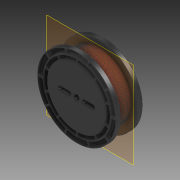
# Autodesk Inventor part: 1240_Wire Spool and Wire
Saved by Autodesk Inventor 2020 (Build 240168000, 168)
## iProperties
Created: 2019-09-24
Part Number: 1240_Wire Spool and Wire
Material: Generic
Document SubType Name: Modeling
Designer: MPI
Density: 1 g/cm^3
Appearance: Default
Author: MPI
Autodesk Inventor part; units mm, degrees
ref_plane "YZ Plane" through (0, 0, 0) normal (1, 0, 0) x (0, 1, 0)
ref_plane "XZ Plane" through (0, 0, 0) normal (0, 1, 0) x (-1, 0, 0)
ref_plane "XY Plane" through (0, 0, 0) normal (0, 0, 1) x (1, 0, 0)
sketch "Sketch1" plane through (0, 0, 0) normal (0, 0, 1) x (1, 0, 0)
  circle A0 centre (0, 0) radius 303
  circle A1 centre (0, 0) radius 20
  line L0 (-125, 15) -> (-57.5, 15)
  line L1 (-57.5, -15) -> (-125, -15)
  line L2 (57.5, 15) -> (125, 15)
  line L3 (125, -15) -> (57.5, -15)
  arc A2 (-57.5, -15) -> (-57.5, 15) centre (-57.5, 0) ccw
  arc A3 (57.5, 15) -> (57.5, -15) centre (57.5, 0) ccw
  arc A4 (125, -15) -> (125, 15) centre (125, 0) ccw
  arc A5 (-125, 15) -> (-125, -15) centre (-125, 0) ccw
  dimension "d0" = 606
  dimension "d12" = 40
  dimension "d15" = 30
  dimension "d16" = 30
  dimension "d17" = 15
  dimension "d18" = 15
  dimension "d19" = 115
  dimension "d20" = 57.5
  dimension "d21" = 250
  dimension "d22" = 125
  constraints: 8 end point, 8 point on circle, 6 centre point, 2 coincident, 2 horizontal, 2 parallel
  measures "d0" diameter of A0
  measures "d12" diameter of A1
  measures "d15" distance of L0.end L1.start
  measures "d16" distance of L3.end L2.start
  measures "d17" distance from line of L3 point (0, 0)
  measures "d18" distance from line of L1 point (0, 0)
  measures "d19" distance of A3.centre A2.centre
  measures "d20" distance of point (0, 0) A2.centre
  measures "d21" distance of A4.centre A5.centre
  measures "d22" distance of point (0, 0) A5.centre
extrude "Extrusion1" add sketch "Sketch1" along normal blind 35
sketch "Sketch2" plane through (0, 0, 35) normal (0, 0, 1) x (1, 0, 0)
  circle A0 centre (0, 0) radius 243
  circle A1 centre (0, 0) radius 20
  arc A2 (-125, 15) -> (-125, -15) centre (-125, 0) ccw projected
  arc A3 (-125, 15) -> (-125, -15) centre (-125, 0) ccw
  arc A4 (-57.5, -15) -> (-57.5, 15) centre (-57.5, 0) ccw projected
  arc A5 (-57.5, -15) -> (-57.5, 15) centre (-57.5, 0) ccw
  arc A6 (57.5, 15) -> (57.5, -15) centre (57.5, 0) ccw projected
  arc A7 (57.5, 15) -> (57.5, -15) centre (57.5, 0) ccw
  arc A8 (125, -15) -> (125, 15) centre (125, 0) ccw projected
  arc A9 (125, -15) -> (125, 15) centre (125, 0) ccw
  line L0 (-125, 15) -> (-57.5, 15) projected
  line L1 (-57.5, -15) -> (-125, -15) projected
  line L2 (-125, 15) -> (-57.5, 15)
  line L3 (-57.5, -15) -> (-125, -15)
  line L4 (125, -15) -> (57.5, -15) projected
  line L5 (57.5, 15) -> (125, 15)
  line L6 (125, -15) -> (57.5, -15)
  point P0 (125, 15)
  dimension "d3" = 486
  dimension "d14" = 40
  constraints: 9 end point, 9 point on circle, 6 centre point, 6 coincident, 2 horizontal, 2 parallel
  measures "d3" diameter of A0
  measures "d14" diameter of A1
extrude "Extrusion2" add sketch "Sketch2" along normal blind 134 separate body
sketch "Sketch3" plane through (0, 0, 169) normal (0, 0, 1) x (1, 0, 0)
  circle A0 centre (0, 0) radius 303
  circle A1 centre (0, 0) radius 20
  arc A2 (-125, 15) -> (-125, -15) centre (-125, 0) ccw projected
  arc A3 (-125, 15) -> (-125, -15) centre (-125, 0) ccw
  arc A4 (-57.5, -15) -> (-57.5, 15) centre (-57.5, 0) ccw projected
  arc A5 (-57.5, -15) -> (-57.5, 15) centre (-57.5, 0) ccw
  arc A6 (57.5, 15) -> (57.5, -15) centre (57.5, 0) ccw projected
  arc A7 (57.5, 15) -> (57.5, -15) centre (57.5, 0) ccw
  arc A8 (125, -15) -> (125, 15) centre (125, 0) ccw projected
  arc A9 (125, -15) -> (125, 15) centre (125, 0) ccw
  line L0 (-57.5, -15) -> (-125, -15) projected
  line L1 (-125, 15) -> (-57.5, 15)
  line L2 (-57.5, -15) -> (-125, -15)
  line L3 (57.5, 15) -> (125, 15) projected
  line L4 (125, -15) -> (57.5, -15) projected
  line L5 (57.5, 15) -> (125, 15)
  line L6 (125, -15) -> (57.5, -15)
  dimension "d6" = 606
  dimension "d13" = 40
  constraints: 10 point on circle, 8 end point, 6 centre point, 6 coincident, 2 horizontal, 2 parallel
  measures "d6" diameter of A0
  measures "d13" diameter of A1
extrude "Extrusion3" add sketch "Sketch3" along normal blind 35 separate body
sketch "Sketch5" plane through (0, 0, 204) normal (0, 0, 1) x (1, 0, 0)
  circle A0 centre (0, 0) radius 303 projected
  line L0 (125, -15) -> (57.5, -15) projected
  arc A1 (57.5, 15) -> (57.5, -15) centre (57.5, 0) ccw projected
  line L1 (57.5, 15) -> (125, 15) projected
  arc A2 (125, -15) -> (125, 15) centre (125, 0) ccw projected
  circle A3 centre (0, 0) radius 20 projected
  line L2 (-125, 15) -> (-57.5, 15) projected
  arc A4 (-57.5, -15) -> (-57.5, 15) centre (-57.5, 0) ccw projected
  line L3 (-57.5, -15) -> (-125, -15) projected
  arc A5 (-125, 15) -> (-125, -15) centre (-125, 0) ccw projected
  circle A6 centre (0, 0) radius 303 projected
  line L4 (0, 0) -> (303, 0) construction
  circle A7 centre (0, 0) radius 20 projected
  line L5 (0, 0) -> (303, 0) construction
  arc A8 (79.7264, 245.3726) -> (-79.7264, 245.3726) centre (0, 0) ccw
  line L6 (0, 0) -> (-6.1803, 19.0211)
  line L7 (-79.7264, 245.3726) -> (-93.6321, 288.1701)
  line L8 (0, 0) -> (6.1803, 19.0211)
  line L9 (79.7264, 245.3726) -> (93.6321, 288.1701)
  arc A9 (93.6321, 288.1701) -> (-93.6321, 288.1701) centre (0, 0) ccw
  line L10 (-87.3188, 284.92) -> (-76.5015, 251.6277)
  arc A10 (76.5015, 251.6277) -> (-76.5015, 251.6277) centre (0, 0) ccw
  line L11 (76.5015, 251.6277) -> (87.3188, 284.92)
  arc A11 (87.3188, 284.92) -> (-87.3188, 284.92) centre (0, 0) ccw
  dimension "d26" = 45
  dimension "d27" = 5
  constraints: 16 end point, 12 point on circle, 4 centre point, 2 collinear, 2 horizontal, 1 concentric, 3 other
  measures "d26" radial gap between concentric circles of A0 A8
  measures "d27" distance between parallel lines of L7 L10
extrude "Extrusion5" cut sketch "Sketch5" against normal blind 30 contours A11 L11 A10 L10 bodies 3
fillet "Fillet1" radius 2 12 edges at (-87.3188, 284.92, 189) (0, 298, 174) (-81.9102, 268.2739, 174) (-76.5015, 251.6277, 189) (0, 263, 174) (87.3188, 284.92, 189) (81.9102, 268.2739, 174) (76.5015, 251.6277, 189) (0, 298, 204) (-81.9102, 268.2739, 204) (0, 263, 204) (81.9102, 268.2739, 204)
pattern_circular "Circular Pattern1" count 10 over 360 about axis through (0, 0, 169) along (0, 0, 1) of "Extrusion5", "Fillet1" bodies 3
sketch "Sketch6" plane through (0, 0, 204) normal (0, 0, 1) x (1, 0, 0)
  arc A0 (246.8073, 170.5466) -> (241.1654, 171.5087) centre (243.5166, 168.2727) ccw projected
  arc A1 (299.9161, 7.0946) -> (246.8073, 170.5466) centre (0, 0) ccw projected
  arc A2 (295.9172, 3) -> (299.9161, 7.0946) centre (295.9172, 7) ccw projected
  line L0 (264.9075, 3) -> (295.9172, 3) projected
  arc A3 (260.9089, 6.8943) -> (264.9075, 3) centre (264.9075, 7) ccw projected
  arc A4 (260.9089, 6.8943) -> (215.1321, 147.7808) centre (0, 0) ccw projected
  arc A5 (216.0781, 153.2817) -> (215.1321, 147.7808) centre (218.4292, 150.0456) ccw projected
  line L1 (241.1654, 171.5087) -> (216.0781, 153.2817) projected
  arc A6 (238.4671, -182.0259) -> (237.6387, -176.3628) centre (235.2876, -179.5989) ccw projected
  arc A7 (99.4265, -283.0448) -> (238.4671, -182.0259) centre (0, 0) ccw projected
  arc A8 (94.2966, -280.5069) -> (99.4265, -283.0448) centre (98.1008, -279.2709) ccw projected
  line L2 (84.7141, -251.015) -> (94.2966, -280.5069) projected
  arc A9 (87.1822, -246.0087) -> (84.7141, -251.015) centre (88.5183, -249.7789) ccw projected
  arc A10 (87.1822, -246.0087) -> (207.0274, -158.9361) centre (0, 0) ccw projected
  arc A11 (212.5513, -158.1358) -> (207.0274, -158.9361) centre (210.2002, -161.3719) ccw projected
  line L3 (237.6387, -176.3628) -> (212.5513, -158.1358) projected
  arc A12 (-99.4265, -283.0448) -> (-94.2966, -280.5069) centre (-98.1008, -279.2709) ccw projected
  arc A13 (-238.4671, -182.0259) -> (-99.4265, -283.0448) centre (0, 0) ccw projected
  arc A14 (-237.6387, -176.3628) -> (-238.4671, -182.0259) centre (-235.2876, -179.5989) ccw projected
  line L4 (-212.5513, -158.1358) -> (-237.6387, -176.3628) projected
  arc A15 (-207.0274, -158.9361) -> (-212.5513, -158.1358) centre (-210.2002, -161.3719) ccw projected
  arc A16 (-207.0274, -158.9361) -> (-87.1822, -246.0087) centre (0, 0) ccw projected
  arc A17 (-84.7141, -251.015) -> (-87.1822, -246.0087) centre (-88.5183, -249.7789) ccw projected
  line L5 (-94.2966, -280.5069) -> (-84.7141, -251.015) projected
  arc A18 (-299.9161, 7.0946) -> (-295.9172, 3) centre (-295.9172, 7) ccw projected
  arc A19 (-246.8073, 170.5466) -> (-299.9161, 7.0946) centre (0, 0) ccw projected
  arc A20 (-241.1654, 171.5087) -> (-246.8073, 170.5466) centre (-243.5166, 168.2727) ccw projected
  line L6 (-216.0781, 153.2817) -> (-241.1654, 171.5087) projected
  arc A21 (-215.1321, 147.7808) -> (-216.0781, 153.2817) centre (-218.4292, 150.0456) ccw projected
  arc A22 (-215.1321, 147.7808) -> (-260.9089, 6.8943) centre (0, 0) ccw projected
  arc A23 (-264.9075, 3) -> (-260.9089, 6.8943) centre (-264.9075, 7) ccw projected
  line L7 (-295.9172, 3) -> (-264.9075, 3) projected
  arc A24 (-85.9318, 287.4295) -> (-88.5903, 282.361) centre (-84.7861, 283.5971) ccw projected
  arc A25 (85.9318, 287.4295) -> (-85.9318, 287.4295) centre (0, 0) ccw projected
  arc A26 (88.5903, 282.361) -> (85.9318, 287.4295) centre (84.7861, 283.5971) ccw projected
  line L8 (79.0078, 252.8691) -> (88.5903, 282.361) projected
  arc A27 (74.0684, 250.2696) -> (79.0078, 252.8691) centre (75.2035, 254.1052) ccw projected
  arc A28 (74.0684, 250.2696) -> (-74.0684, 250.2696) centre (0, 0) ccw projected
  arc A29 (-79.0078, 252.8691) -> (-74.0684, 250.2696) centre (-75.2035, 254.1052) ccw projected
  line L9 (-88.5903, 282.361) -> (-79.0078, 252.8691) projected
  circle A30 centre (0, 0) radius 303 projected
  line L10 (125, -15) -> (57.5, -15) projected
  arc A31 (57.5, 15) -> (57.5, -15) centre (57.5, 0) ccw projected
  line L11 (57.5, 15) -> (125, 15) projected
  arc A32 (125, -15) -> (125, 15) centre (125, 0) ccw projected
  circle A33 centre (0, 0) radius 20 projected
  line L12 (-125, 15) -> (-57.5, 15) projected
  arc A34 (-57.5, -15) -> (-57.5, 15) centre (-57.5, 0) ccw projected
  line L13 (-57.5, -15) -> (-125, -15) projected
  arc A35 (-125, 15) -> (-125, -15) centre (-125, 0) ccw projected
  arc A36 (-238.4671, 182.0259) -> (-237.6387, 176.3628) centre (-235.2876, 179.5989) ccw projected
  arc A37 (-99.4265, 283.0448) -> (-238.4671, 182.0259) centre (0, 0) ccw projected
  arc A38 (-94.2966, 280.5069) -> (-99.4265, 283.0448) centre (-98.1008, 279.2709) ccw projected
  line L14 (-84.7141, 251.015) -> (-94.2966, 280.5069) projected
  arc A39 (-87.1822, 246.0087) -> (-84.7141, 251.015) centre (-88.5183, 249.7789) ccw projected
  arc A40 (-87.1822, 246.0087) -> (-207.0274, 158.9361) centre (0, 0) ccw projected
  arc A41 (-212.5513, 158.1358) -> (-207.0274, 158.9361) centre (-210.2002, 161.3719) ccw projected
  line L15 (-237.6387, 176.3628) -> (-212.5513, 158.1358) projected
  arc A42 (-246.8073, -170.5466) -> (-241.1654, -171.5087) centre (-243.5166, -168.2727) ccw projected
  arc A43 (-299.9161, -7.0946) -> (-246.8073, -170.5466) centre (0, 0) ccw projected
  arc A44 (-295.9172, -3) -> (-299.9161, -7.0946) centre (-295.9172, -7) ccw projected
  line L16 (-264.9075, -3) -> (-295.9172, -3) projected
  arc A45 (-260.9089, -6.8943) -> (-264.9075, -3) centre (-264.9075, -7) ccw projected
  arc A46 (-260.9089, -6.8943) -> (-215.1321, -147.7808) centre (0, 0) ccw projected
  arc A47 (-216.0781, -153.2817) -> (-215.1321, -147.7808) centre (-218.4292, -150.0456) ccw projected
  line L17 (-241.1654, -171.5087) -> (-216.0781, -153.2817) projected
  arc A48 (85.9318, -287.4295) -> (88.5903, -282.361) centre (84.7861, -283.5971) ccw projected
  arc A49 (-85.9318, -287.4295) -> (85.9318, -287.4295) centre (0, 0) ccw projected
  arc A50 (-88.5903, -282.361) -> (-85.9318, -287.4295) centre (-84.7861, -283.5971) ccw projected
  line L18 (-79.0078, -252.8691) -> (-88.5903, -282.361) projected
  arc A51 (-74.0684, -250.2696) -> (-79.0078, -252.8691) centre (-75.2035, -254.1052) ccw projected
  arc A52 (-74.0684, -250.2696) -> (74.0684, -250.2696) centre (0, 0) ccw projected
  arc A53 (79.0078, -252.8691) -> (74.0684, -250.2696) centre (75.2035, -254.1052) ccw projected
  line L19 (88.5903, -282.361) -> (79.0078, -252.8691) projected
  arc A54 (299.9161, -7.0946) -> (295.9172, -3) centre (295.9172, -7) ccw projected
  arc A55 (246.8073, -170.5466) -> (299.9161, -7.0946) centre (0, 0) ccw projected
  arc A56 (241.1654, -171.5087) -> (246.8073, -170.5466) centre (243.5166, -168.2727) ccw projected
  line L20 (216.0781, -153.2817) -> (241.1654, -171.5087) projected
  arc A57 (215.1321, -147.7808) -> (216.0781, -153.2817) centre (218.4292, -150.0456) ccw projected
  arc A58 (215.1321, -147.7808) -> (260.9089, -6.8943) centre (0, 0) ccw projected
  arc A59 (264.9075, -3) -> (260.9089, -6.8943) centre (264.9075, -7) ccw projected
  line L21 (295.9172, -3) -> (264.9075, -3) projected
  arc A60 (99.4265, 283.0448) -> (94.2966, 280.5069) centre (98.1008, 279.2709) ccw projected
  arc A61 (238.4671, 182.0259) -> (99.4265, 283.0448) centre (0, 0) ccw projected
  arc A62 (237.6387, 176.3628) -> (238.4671, 182.0259) centre (235.2876, 179.5989) ccw projected
  line L22 (212.5513, 158.1358) -> (237.6387, 176.3628) projected
  arc A63 (207.0274, 158.9361) -> (212.5513, 158.1358) centre (210.2002, 161.3719) ccw projected
  arc A64 (207.0274, 158.9361) -> (87.1822, 246.0087) centre (0, 0) ccw projected
  arc A65 (84.7141, 251.015) -> (87.1822, 246.0087) centre (88.5183, 249.7789) ccw projected
  line L23 (94.2966, 280.5069) -> (84.7141, 251.015) projected
  arc A66 (207.0274, 158.9361) -> (87.1822, 246.0087) centre (0, 0) ccw projected
  arc A67 (147.9789, 208.8977) -> (3.0695, 255.9816) centre (0, 0) ccw
  circle A68 centre (0, 0) radius 20 projected
  arc A69 (130.4615, 184.5422) -> (2.9256, 225.9811) centre (0, 0) ccw
  line L24 (0, 0) -> (0, 20)
  line L25 (2.9256, 225.9811) -> (3.0695, 255.9816)
  line L26 (0, 0) -> (11.7557, 16.1803)
  line L27 (130.4615, 184.5422) -> (147.9789, 208.8977)
  line L28 (5.0598, 253.9496) -> (4.9351, 227.9466)
  arc A70 (129.9911, 187.3134) -> (4.9351, 227.9466) centre (0, 0) ccw
  line L29 (129.9911, 187.3134) -> (145.1744, 208.4236)
  arc A71 (145.1744, 208.4236) -> (5.0598, 253.9496) centre (0, 0) ccw
  dimension "d34" = 30
  dimension "d35" = 5
  dimension "d39" = 2
  constraints: 12 end point, 10 point on circle, 4 centre point, 2 coincident, 3 other
  measures "d34" radial gap between concentric circles of A67 A69
  measures "d35" radial gap between concentric circles of A28 A67
  measures "d39" radial gap between concentric circles of A67 A71
extrude "Extrusion6" cut sketch "Sketch6" against normal blind 30 contours A71 L29 A70 L28 bodies 3
fillet "Fillet3" radius 2 12 edges at (4.9974, 240.9481, 174) (5.0598, 253.9496, 189) (78.4903, 241.5684, 174) (78.4903, 241.5684, 204) (4.9974, 240.9481, 204) (70.4559, 216.8409, 204) (4.9351, 227.9466, 189) (129.9911, 187.3134, 189) (137.5827, 197.8685, 204) (70.4559, 216.8409, 174) (137.5827, 197.8685, 174) (145.1744, 208.4236, 189)
pattern_circular "Circular Pattern2" count 10 over 360 about axis through (0, 0, 169) along (0, 0, 1) of "Fillet3", "Extrusion6" bodies 3
fillet "Fillet4" radius 2 22 edges at (-303, 0, 35) (-303, 0, 0) (91.25, 15, 0) (140, 0, 0) (91.25, -15, 0) (42.5, 0, 0) (-20, 0, 0) (-91.25, -15, 0) (-140, 0, 0) (-91.25, 15, 0) (-42.5, 0, 0) (-303, 0, 204) (-303, 0, 169) (-91.25, -15, 204) (-140, 0, 204) (-91.25, 15, 204) (-42.5, 0, 204) (-20, 0, 204) (42.5, 0, 204) (91.25, 15, 204) (140, 0, 204) (91.25, -15, 204)
sketch "Sketch7" plane through (0, 0, 0) normal (0, 0, -1) x (-1, 0, 0)
  point P0 (0, 0)
sketch "Sketch8" plane through (0, 0, 0) normal (0, 0, -1) x (-1, 0, 0)
  arc A0 (-4.9351, 227.9466) -> (-129.9911, 187.3134) centre (0, 0) ccw projected
  line L0 (-5.0598, 253.9496) -> (-4.9351, 227.9466) projected
  arc A1 (-5.0598, 253.9496) -> (-145.1744, 208.4236) centre (0, 0) ccw projected
  line L1 (-129.9911, 187.3134) -> (-145.1744, 208.4236) projected
  arc A2 (76.5015, 251.6277) -> (-76.5015, 251.6277) centre (0, 0) ccw projected
  line L2 (-76.5015, 251.6277) -> (-87.3188, 284.92) projected
  arc A3 (87.3188, 284.92) -> (-87.3188, 284.92) centre (0, 0) ccw projected
  line L3 (87.3188, 284.92) -> (76.5015, 251.6277) projected
extrude "Extrusion7" cut sketch "Sketch8" against normal blind 30 bodies 1
fillet "Fillet5" radius 2 24 edges at (76.5015, 251.6277, 15) (81.9102, 268.2739, 0) (0, 263, 0) (145.1744, 208.4236, 15) (78.4903, 241.5684, 0) (137.5827, 197.8685, 0) (70.4559, 216.8409, 0) (137.5827, 197.8685, 30) (70.4559, 216.8409, 30) (0, 263, 30) (0, 298, 0) (81.9102, 268.2739, 30) (0, 298, 30) (-81.9102, 268.2739, 30) (-81.9102, 268.2739, 0) (4.9974, 240.9481, 0) (-87.3188, 284.92, 15) (-76.5015, 251.6277, 15) (87.3188, 284.92, 15) (129.9911, 187.3134, 15) (4.9351, 227.9466, 15) (4.9974, 240.9481, 30) (5.0598, 253.9496, 15) (78.4903, 241.5684, 30)
pattern_circular "Circular Pattern3" count 10 over 360 about axis through (0, 0, 0) along (0, 0, 1) of "Extrusion7", "Fillet5" bodies 1
sketch "Sketch9" plane through (0, 0, 0) normal (1, 0, 0) x (0, 1, 0)
  line L0 (243, 35) -> (243, 169) projected
  line L1 (-243, 35) -> (-243, 169) projected
  line L2 (243, 102) -> (-243, 102)
  line L3 (0, 102) -> (0, 0)
  line L4 (243.5, 169) -> (248.5, 169)
  line L5 (249, 168.5) -> (249, 163.5)
  line L6 (248.5, 163) -> (243.5, 163)
  line L7 (243, 163.5) -> (243, 168.5)
  arc A0 (249, 168.5) -> (248.5, 169) centre (248.5, 168.5) ccw
  arc A1 (248.5, 163) -> (249, 163.5) centre (248.5, 163.5) ccw
  arc A2 (243, 163.5) -> (243.5, 163) centre (243.5, 163.5) ccw
  arc A3 (243.5, 169) -> (243, 168.5) centre (243.5, 168.5) ccw
  line L8 (248.5, 156.91) -> (243.5, 156.91)
  arc A4 (243, 157.41) -> (243.5, 156.91) centre (243.5, 157.41) ccw
  line L9 (243, 157.41) -> (243, 162.41)
  arc A5 (243.5, 162.91) -> (243, 162.41) centre (243.5, 162.41) ccw
  line L10 (243.5, 162.91) -> (248.5, 162.91)
  line L11 (249, 162.41) -> (249, 157.41)
  arc A6 (248.5, 156.91) -> (249, 157.41) centre (248.5, 157.41) ccw
  arc A7 (249, 162.41) -> (248.5, 162.91) centre (248.5, 162.41) ccw
  line L12 (248.5, 150.82) -> (243.5, 150.82)
  arc A8 (243, 151.32) -> (243.5, 150.82) centre (243.5, 151.32) ccw
  line L13 (243, 151.32) -> (243, 156.32)
  arc A9 (243.5, 156.82) -> (243, 156.32) centre (243.5, 156.32) ccw
  line L14 (243.5, 156.82) -> (248.5, 156.82)
  line L15 (249, 156.32) -> (249, 151.32)
  arc A10 (248.5, 150.82) -> (249, 151.32) centre (248.5, 151.32) ccw
  arc A11 (249, 156.32) -> (248.5, 156.82) centre (248.5, 156.32) ccw
  line L16 (248.5, 144.73) -> (243.5, 144.73)
  arc A12 (243, 145.23) -> (243.5, 144.73) centre (243.5, 145.23) ccw
  line L17 (243, 145.23) -> (243, 150.23)
  arc A13 (243.5, 150.73) -> (243, 150.23) centre (243.5, 150.23) ccw
  line L18 (243.5, 150.73) -> (248.5, 150.73)
  line L19 (249, 150.23) -> (249, 145.23)
  arc A14 (248.5, 144.73) -> (249, 145.23) centre (248.5, 145.23) ccw
  arc A15 (249, 150.23) -> (248.5, 150.73) centre (248.5, 150.23) ccw
  line L20 (248.5, 138.64) -> (243.5, 138.64)
  arc A16 (243, 139.14) -> (243.5, 138.64) centre (243.5, 139.14) ccw
  line L21 (243, 139.14) -> (243, 144.14)
  arc A17 (243.5, 144.64) -> (243, 144.14) centre (243.5, 144.14) ccw
  line L22 (243.5, 144.64) -> (248.5, 144.64)
  line L23 (249, 144.14) -> (249, 139.14)
  arc A18 (248.5, 138.64) -> (249, 139.14) centre (248.5, 139.14) ccw
  arc A19 (249, 144.14) -> (248.5, 144.64) centre (248.5, 144.14) ccw
  line L24 (248.5, 132.55) -> (243.5, 132.55)
  arc A20 (243, 133.05) -> (243.5, 132.55) centre (243.5, 133.05) ccw
  line L25 (243, 133.05) -> (243, 138.05)
  arc A21 (243.5, 138.55) -> (243, 138.05) centre (243.5, 138.05) ccw
  line L26 (243.5, 138.55) -> (248.5, 138.55)
  line L27 (249, 138.05) -> (249, 133.05)
  arc A22 (248.5, 132.55) -> (249, 133.05) centre (248.5, 133.05) ccw
  arc A23 (249, 138.05) -> (248.5, 138.55) centre (248.5, 138.05) ccw
  line L28 (248.5, 126.46) -> (243.5, 126.46)
  arc A24 (243, 126.96) -> (243.5, 126.46) centre (243.5, 126.96) ccw
  line L29 (243, 126.96) -> (243, 131.96)
  arc A25 (243.5, 132.46) -> (243, 131.96) centre (243.5, 131.96) ccw
  line L30 (243.5, 132.46) -> (248.5, 132.46)
  line L31 (249, 131.96) -> (249, 126.96)
  arc A26 (248.5, 126.46) -> (249, 126.96) centre (248.5, 126.96) ccw
  arc A27 (249, 131.96) -> (248.5, 132.46) centre (248.5, 131.96) ccw
  line L32 (248.5, 120.37) -> (243.5, 120.37)
  arc A28 (243, 120.87) -> (243.5, 120.37) centre (243.5, 120.87) ccw
  line L33 (243, 120.87) -> (243, 125.87)
  arc A29 (243.5, 126.37) -> (243, 125.87) centre (243.5, 125.87) ccw
  line L34 (243.5, 126.37) -> (248.5, 126.37)
  line L35 (249, 125.87) -> (249, 120.87)
  arc A30 (248.5, 120.37) -> (249, 120.87) centre (248.5, 120.87) ccw
  arc A31 (249, 125.87) -> (248.5, 126.37) centre (248.5, 125.87) ccw
  line L36 (248.5, 114.28) -> (243.5, 114.28)
  arc A32 (243, 114.78) -> (243.5, 114.28) centre (243.5, 114.78) ccw
  line L37 (243, 114.78) -> (243, 119.78)
  arc A33 (243.5, 120.28) -> (243, 119.78) centre (243.5, 119.78) ccw
  line L38 (243.5, 120.28) -> (248.5, 120.28)
  line L39 (249, 119.78) -> (249, 114.78)
  arc A34 (248.5, 114.28) -> (249, 114.78) centre (248.5, 114.78) ccw
  arc A35 (249, 119.78) -> (248.5, 120.28) centre (248.5, 119.78) ccw
  line L40 (248.5, 108.19) -> (243.5, 108.19)
  arc A36 (243, 108.69) -> (243.5, 108.19) centre (243.5, 108.69) ccw
  line L41 (243, 108.69) -> (243, 113.69)
  arc A37 (243.5, 114.19) -> (243, 113.69) centre (243.5, 113.69) ccw
  line L42 (243.5, 114.19) -> (248.5, 114.19)
  line L43 (249, 113.69) -> (249, 108.69)
  arc A38 (248.5, 108.19) -> (249, 108.69) centre (248.5, 108.69) ccw
  arc A39 (249, 113.69) -> (248.5, 114.19) centre (248.5, 113.69) ccw
  line L44 (248.5, 102.1) -> (243.5, 102.1)
  arc A40 (243, 102.6) -> (243.5, 102.1) centre (243.5, 102.6) ccw
  line L45 (243, 102.6) -> (243, 107.6)
  arc A41 (243.5, 108.1) -> (243, 107.6) centre (243.5, 107.6) ccw
  line L46 (243.5, 108.1) -> (248.5, 108.1)
  line L47 (249, 107.6) -> (249, 102.6)
  arc A42 (248.5, 102.1) -> (249, 102.6) centre (248.5, 102.6) ccw
  arc A43 (249, 107.6) -> (248.5, 108.1) centre (248.5, 107.6) ccw
  line L48 (248.5, 96.01) -> (243.5, 96.01)
  arc A44 (243, 96.51) -> (243.5, 96.01) centre (243.5, 96.51) ccw
  line L49 (243, 96.51) -> (243, 101.51)
  arc A45 (243.5, 102.01) -> (243, 101.51) centre (243.5, 101.51) ccw
  line L50 (243.5, 102.01) -> (248.5, 102.01)
  line L51 (249, 101.51) -> (249, 96.51)
  arc A46 (248.5, 96.01) -> (249, 96.51) centre (248.5, 96.51) ccw
  arc A47 (249, 101.51) -> (248.5, 102.01) centre (248.5, 101.51) ccw
  line L52 (248.5, 89.92) -> (243.5, 89.92)
  arc A48 (243, 90.42) -> (243.5, 89.92) centre (243.5, 90.42) ccw
  line L53 (243, 90.42) -> (243, 95.42)
  arc A49 (243.5, 95.92) -> (243, 95.42) centre (243.5, 95.42) ccw
  line L54 (243.5, 95.92) -> (248.5, 95.92)
  line L55 (249, 95.42) -> (249, 90.42)
  arc A50 (248.5, 89.92) -> (249, 90.42) centre (248.5, 90.42) ccw
  arc A51 (249, 95.42) -> (248.5, 95.92) centre (248.5, 95.42) ccw
  line L56 (248.5, 83.83) -> (243.5, 83.83)
  arc A52 (243, 84.33) -> (243.5, 83.83) centre (243.5, 84.33) ccw
  line L57 (243, 84.33) -> (243, 89.33)
  arc A53 (243.5, 89.83) -> (243, 89.33) centre (243.5, 89.33) ccw
  line L58 (243.5, 89.83) -> (248.5, 89.83)
  line L59 (249, 89.33) -> (249, 84.33)
  arc A54 (248.5, 83.83) -> (249, 84.33) centre (248.5, 84.33) ccw
  arc A55 (249, 89.33) -> (248.5, 89.83) centre (248.5, 89.33) ccw
  line L60 (248.5, 77.74) -> (243.5, 77.74)
  arc A56 (243, 78.24) -> (243.5, 77.74) centre (243.5, 78.24) ccw
  line L61 (243, 78.24) -> (243, 83.24)
  arc A57 (243.5, 83.74) -> (243, 83.24) centre (243.5, 83.24) ccw
  line L62 (243.5, 83.74) -> (248.5, 83.74)
  line L63 (249, 83.24) -> (249, 78.24)
  arc A58 (248.5, 77.74) -> (249, 78.24) centre (248.5, 78.24) ccw
  arc A59 (249, 83.24) -> (248.5, 83.74) centre (248.5, 83.24) ccw
  line L64 (248.5, 71.65) -> (243.5, 71.65)
  arc A60 (243, 72.15) -> (243.5, 71.65) centre (243.5, 72.15) ccw
  line L65 (243, 72.15) -> (243, 77.15)
  arc A61 (243.5, 77.65) -> (243, 77.15) centre (243.5, 77.15) ccw
  line L66 (243.5, 77.65) -> (248.5, 77.65)
  line L67 (249, 77.15) -> (249, 72.15)
  arc A62 (248.5, 71.65) -> (249, 72.15) centre (248.5, 72.15) ccw
  arc A63 (249, 77.15) -> (248.5, 77.65) centre (248.5, 77.15) ccw
  line L68 (248.5, 65.56) -> (243.5, 65.56)
  arc A64 (243, 66.06) -> (243.5, 65.56) centre (243.5, 66.06) ccw
  line L69 (243, 66.06) -> (243, 71.06)
  arc A65 (243.5, 71.56) -> (243, 71.06) centre (243.5, 71.06) ccw
  line L70 (243.5, 71.56) -> (248.5, 71.56)
  line L71 (249, 71.06) -> (249, 66.06)
  arc A66 (248.5, 65.56) -> (249, 66.06) centre (248.5, 66.06) ccw
  arc A67 (249, 71.06) -> (248.5, 71.56) centre (248.5, 71.06) ccw
  line L72 (248.5, 59.47) -> (243.5, 59.47)
  arc A68 (243, 59.97) -> (243.5, 59.47) centre (243.5, 59.97) ccw
  line L73 (243, 59.97) -> (243, 64.97)
  arc A69 (243.5, 65.47) -> (243, 64.97) centre (243.5, 64.97) ccw
  line L74 (243.5, 65.47) -> (248.5, 65.47)
  line L75 (249, 64.97) -> (249, 59.97)
  arc A70 (248.5, 59.47) -> (249, 59.97) centre (248.5, 59.97) ccw
  arc A71 (249, 64.97) -> (248.5, 65.47) centre (248.5, 64.97) ccw
  line L76 (248.5, 53.38) -> (243.5, 53.38)
  arc A72 (243, 53.88) -> (243.5, 53.38) centre (243.5, 53.88) ccw
  line L77 (243, 53.88) -> (243, 58.88)
  arc A73 (243.5, 59.38) -> (243, 58.88) centre (243.5, 58.88) ccw
  line L78 (243.5, 59.38) -> (248.5, 59.38)
  line L79 (249, 58.88) -> (249, 53.88)
  arc A74 (248.5, 53.38) -> (249, 53.88) centre (248.5, 53.88) ccw
  arc A75 (249, 58.88) -> (248.5, 59.38) centre (248.5, 58.88) ccw
  line L80 (248.5, 47.29) -> (243.5, 47.29)
  arc A76 (243, 47.79) -> (243.5, 47.29) centre (243.5, 47.79) ccw
  line L81 (243, 47.79) -> (243, 52.79)
  arc A77 (243.5, 53.29) -> (243, 52.79) centre (243.5, 52.79) ccw
  line L82 (243.5, 53.29) -> (248.5, 53.29)
  line L83 (249, 52.79) -> (249, 47.79)
  arc A78 (248.5, 47.29) -> (249, 47.79) centre (248.5, 47.79) ccw
  arc A79 (249, 52.79) -> (248.5, 53.29) centre (248.5, 52.79) ccw
  line L84 (248.5, 41.2) -> (243.5, 41.2)
  arc A80 (243, 41.7) -> (243.5, 41.2) centre (243.5, 41.7) ccw
  line L85 (243, 41.7) -> (243, 46.7)
  arc A81 (243.5, 47.2) -> (243, 46.7) centre (243.5, 46.7) ccw
  line L86 (243.5, 47.2) -> (248.5, 47.2)
  line L87 (249, 46.7) -> (249, 41.7)
  arc A82 (248.5, 41.2) -> (249, 41.7) centre (248.5, 41.7) ccw
  arc A83 (249, 46.7) -> (248.5, 47.2) centre (248.5, 46.7) ccw
  line L88 (248.5, 35.11) -> (243.5, 35.11)
  arc A84 (243, 35.61) -> (243.5, 35.11) centre (243.5, 35.61) ccw
  line L89 (243, 35.61) -> (243, 40.61)
  arc A85 (243.5, 41.11) -> (243, 40.61) centre (243.5, 40.61) ccw
  line L90 (243.5, 41.11) -> (248.5, 41.11)
  line L91 (249, 40.61) -> (249, 35.61)
  arc A86 (248.5, 35.11) -> (249, 35.61) centre (248.5, 35.61) ccw
  arc A87 (249, 40.61) -> (248.5, 41.11) centre (248.5, 40.61) ccw
  point P0 (249, 163)
  point P1 (249, 169)
  point P2 (243, 163)
  point P3 (249, 156.91)
  point P4 (243, 156.91)
  point P5 (243, 162.91)
  point P6 (249, 162.91)
  point P7 (249, 150.82)
  point P8 (243, 150.82)
  point P9 (243, 156.82)
  point P10 (249, 156.82)
  point P11 (249, 144.73)
  point P12 (243, 144.73)
  point P13 (243, 150.73)
  point P14 (249, 150.73)
  point P15 (249, 138.64)
  point P16 (243, 138.64)
  point P17 (243, 144.64)
  point P18 (249, 144.64)
  point P19 (249, 132.55)
  point P20 (243, 132.55)
  point P21 (243, 138.55)
  point P22 (249, 138.55)
  point P23 (249, 126.46)
  point P24 (243, 126.46)
  point P25 (243, 132.46)
  point P26 (249, 132.46)
  point P27 (249, 120.37)
  point P28 (243, 120.37)
  point P29 (243, 126.37)
  point P30 (249, 126.37)
  point P31 (249, 114.28)
  point P32 (243, 114.28)
  point P33 (243, 120.28)
  point P34 (249, 120.28)
  point P35 (249, 108.19)
  point P36 (243, 108.19)
  point P37 (243, 114.19)
  point P38 (249, 114.19)
  point P39 (249, 102.1)
  point P40 (243, 102.1)
  point P41 (243, 108.1)
  point P42 (249, 108.1)
  point P43 (249, 96.01)
  point P44 (243, 96.01)
  point P45 (243, 102.01)
  point P46 (249, 102.01)
  point P47 (249, 89.92)
  point P48 (243, 89.92)
  point P49 (243, 95.92)
  point P50 (249, 95.92)
  point P51 (249, 83.83)
  point P52 (243, 83.83)
  point P53 (243, 89.83)
  point P54 (249, 89.83)
  point P55 (249, 77.74)
  point P56 (243, 77.74)
  point P57 (243, 83.74)
  point P58 (249, 83.74)
  point P59 (249, 71.65)
  point P60 (243, 71.65)
  point P61 (243, 77.65)
  point P62 (249, 77.65)
  point P63 (249, 65.56)
  point P64 (243, 65.56)
  point P65 (243, 71.56)
  point P66 (249, 71.56)
  point P67 (249, 59.47)
  point P68 (243, 59.47)
  point P69 (243, 65.47)
  point P70 (249, 65.47)
  point P71 (249, 53.38)
  point P72 (243, 53.38)
  point P73 (243, 59.38)
  point P74 (249, 59.38)
  point P75 (249, 47.29)
  point P76 (243, 47.29)
  point P77 (243, 53.29)
  point P78 (249, 53.29)
  point P79 (249, 41.2)
  point P80 (243, 41.2)
  point P81 (243, 47.2)
  point P82 (249, 47.2)
  point P83 (249, 35.11)
  point P84 (243, 35.11)
  point P85 (243, 41.11)
  point P86 (249, 41.11)
  dimension "d51" = 6
  dimension "d52" = 6
  dimension "d53" = 0.5
  dimension "d56" = 6.09
  constraints: 336 vertical alignment, 180 end point, 176 point on circle, 176 point on line, 88 centre point, 87 equal radius, 44 parallel, 42 collinear, 8 tangent, 2 midpoint, 1 horizontal, 1 perpendicular, 1 vertical, 2 other
  measures "d51" distance of point (249, 163) point (243, 163)
  measures "d52" distance of point (249, 169) point (249, 163)
  measures "d53" radius of A0
  measures "d56" distance of L6.start L8.start
revolve "Revolution1" add sketch "Sketch9" angle 360 about axis through (0, 0, 102) along (0, 0, -1) separate body
ref_plane "Work Plane2" through (0, 0, 102) normal (0, 0, 1) x (1, 0, 0)
body "Solid1"
body "Solid2"
body "Solid3"
body "Solid4"
